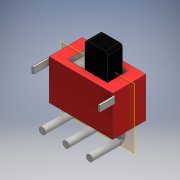
# Autodesk Inventor part: 5MS1S102AM6QE
Saved by Autodesk Inventor 2016 (Build 200138000, 138)
## iProperties
Created: 2018-08-01
Part Number: 5MS1S102AM6QE
Material: Generic
Document SubType Name: Modeling
Designer: Luke
Density: 1 g/cm^3
Appearance: Default
Author: Luke
Autodesk Inventor part; units mm, degrees
ref_plane "YZ Plane" through (0, 0, 0) normal (1, 0, 0) x (0, 1, 0)
sketch "Sketch1" plane through (0, 0, 0) normal (0, 0, 1) x (1, 0, 0)
  line L0 (0, 0) -> (12.7, 0)
  line L1 (12.7, 0) -> (12.7, 6.6)
  line L2 (12.7, 6.6) -> (0, 6.6)
  line L3 (0, 6.6) -> (0, 0)
  dimension "d0" = 12.7
  dimension "d1" = 6.6
  constraints: 8 end point, 2 parallel, 1 horizontal, 1 perpendicular
  measures "d0" distance of L1.end L2.end
  measures "d1" distance of L0.end L1.end
extrude "Extrusion1" add sketch "Sketch1" along normal blind 8
sketch "Sketch2" plane through (0, 0, 0) normal (0, -1, 0) x (1, 0, 0)
  line L0 (0, 0) -> (12.7, 0) construction
  line L1 (12.7, 0) -> (12.7, 8) construction
  line L2 (0, 8) -> (12.7, 8) construction
  line L3 (0, 0) -> (0, 8) construction
  line L4 (0, 0) -> (12.7, 0) construction
  line L5 (6.35, 0) -> (6.35, 8) construction
  line L6 (0, 8) -> (12.7, 8) construction
  line L7 (13.135, 7.585) -> (12.775, 7.585)
  line L8 (12.775, 7.585) -> (12.775, 6.415)
  line L9 (12.775, 6.415) -> (13.135, 6.415)
  line L10 (13.135, 6.415) -> (13.135, 7.585)
  line L11 (13.135, 7.585) -> (12.775, 6.415) construction
  line L12 (12.775, 7.585) -> (13.135, 6.415) construction
  circle A0 centre (6.35, -2.53) radius 0.635
  circle A1 centre (11.05, -2.53) radius 0.635
  circle A2 centre (1.65, -2.53) radius 0.635
  line L13 (11.05, -2.53) -> (6.35, -2.53) construction
  line L14 (6.35, -2.53) -> (1.65, -2.53) construction
  line L15 (-0.435, 7.585) -> (-0.075, 7.585)
  line L16 (-0.075, 7.585) -> (-0.075, 6.415)
  line L17 (-0.075, 6.415) -> (-0.435, 6.415)
  line L18 (-0.435, 6.415) -> (-0.435, 7.585)
  point P0 (12.955, 7)
  dimension "d4" = 1.17
  dimension "d5" = 0.36
  dimension "d6" = 6.605
  dimension "d7" = 1.27
  dimension "d8" = 1.27
  dimension "d9" = 1.27
  dimension "d10" = 9.53
  dimension "d11" = 4.7
  dimension "d12" = 4.7
  dimension "d13" = 1
  constraints: 26 end point, 4 midpoint, 4 symmetric about line, 3 centre point, 3 equal length, 2 horizontal, 1 perpendicular, 1 point on line
  measures "d4" distance of L9.end L7.start
  measures "d5" distance of L8.end L9.end
  measures "d6" distance from line of L5 point (12.955, 7)
  measures "d7" diameter of A0
  measures "d8" diameter of A1
  measures "d9" diameter of A2
  measures "d10" vertical distance of point (12.955, 7) L13.start
  measures "d11" distance of L13.end L13.start
  measures "d12" distance of L14.end L13.end
  measures "d13" distance from line of L2 point (12.955, 7)
extrude "Extrusion2" add sketch "Sketch2" along normal blind 3
ref_plane "Work Plane1" through (0, 2.6, 0) normal (0, 1, 0) x (1, 0, 0)
sketch "Sketch3" plane through (11.05, 0, -2.53) normal (0, 1, 0) x (1, 0, 0)
  circle A0 centre (0, 0) radius 0.635 projected
  circle A1 centre (-4.7, 0) radius 0.635 projected
  circle A2 centre (-9.4, 0) radius 0.635 projected
  point P0 (-11.05, -2.53)
extrude "Extrusion3" add sketch "Sketch3" along normal up to surface (2.6 mm away)
sketch "Sketch4" plane through (0, 0, 0) normal (0, 0, -1) x (-1, 0, 0)
  line L0 (-6.985, 2.6) -> (-5.715, 2.6) projected
  line L1 (-6.35, 2.6) -> (-6.35, 3.235) construction
  circle A0 centre (-6.35, 3.235) radius 0.635
  point P0 (0, 0)
  dimension "d19" = 0.635
  constraints: 2 end point, 1 coincident, 1 midpoint, 1 vertical, 1 vertical alignment, 2 other
  measures "d19" distance of L1.start L1.end
extrude "Extrusion4" add sketch "Sketch4" along normal blind 1.895
sketch "Sketch5" plane through (0, 0, -1.895) normal (0, 0, -1) x (-1, 0, 0)
  arc A0 (-5.715, 3.235) -> (-6.35, 2.6) centre (-6.35, 3.235) ccw construction
  arc A1 (-5.715, 3.235) -> (-6.35, 2.6) centre (-6.35, 3.235) ccw projected
  arc A2 (-6.35, 2.6) -> (-5.715, 3.235) centre (-6.35, 3.235) ccw projected
  point P0 (0, 0)
  constraints: 1 coincident
ref_plane "Work Plane2" through (6.35, 3.235, -1.895) normal (1, 0, 0) x (0, 0, -1)
sketch "Sketch6" plane through (6.35, 3.235, -1.895) normal (1, 0, 0) x (0, 0, -1)
  line L0 (0.635, -0.635) -> (0, -0.635) construction
  line L1 (0, -0.635) -> (0.635, -0.635) construction
  line L2 (0, -0.635) -> (0, 0) construction
  arc A0 (0.635, -0.635) -> (0, 0) centre (0, -0.635) ccw
  point P0 (-1.895, -3.235)
  constraints: 2 point on circle, 1 centre point, 1 coincident
sweep "Sweep1" add profiles "Sketch5" path "Sketch6"
pattern_linear "Rectangular Pattern1" count 3 spacing 4.7 along (-1, 0, 0) of "Sweep1", "Extrusion4" first direction both ways yes
sketch "Sketch7" plane through (-0.435, 0, 7.585) normal (0, 0, 1) x (1, 0, 0)
  line L0 (0.36, 0) -> (0, 0) projected
  line L1 (0.435, 0) -> (13.135, 0) projected
  line L2 (13.135, 0) -> (13.135, 6.6) projected
  line L3 (13.135, 6.6) -> (0.435, 6.6) projected
  line L4 (0.435, 6.6) -> (0.435, 0) projected
  line L5 (0.36, 0) -> (0.36, -3) projected
  line L6 (0.36, 0) -> (0.435, 0)
  line L7 (0, 0) -> (0.435, 0.2)
  line L8 (0.435, 6.6) -> (0.435, 0) projected
  dimension "d27" = 0.2
  constraints: 4 end point, 1 perpendicular, 1 point on line
  measures "d27" distance of L8.end L7.end
extrude "Extrusion5" add sketch "Sketch7" against normal up to surface (1.17 mm away) contours L0 L7 L4 L6
mirror "Mirror1" about plane through (6.35, 3.235, -1.895) normal (1, 0, 0) of "Extrusion5"
ref_plane "Work Plane3" through (0, 3.3, 0) normal (0, -1, 0) x (1, 0, 0)
sketch "Sketch9" plane through (0, 0, 8) normal (0, 0, 1) x (1, 0, 0)
  line L0 (15.849, 3.3) -> (-3.149, 3.3) projected
  line L1 (2.35, 5.3) -> (10.35, 5.3)
  line L2 (10.35, 5.3) -> (10.35, 1.3)
  line L3 (10.35, 1.3) -> (2.35, 1.3)
  line L4 (2.35, 1.3) -> (2.35, 5.3)
  line L5 (0, 0) -> (12.7, 0) construction
  line L6 (12.7, 0) -> (12.7, 6.6) construction
  line L7 (12.7, 6.6) -> (0, 6.6) construction
  line L8 (0, 6.6) -> (0, 0) construction
  line L9 (12.7, 6.6) -> (0, 6.6) construction
  line L10 (6.35, 6.6) -> (6.35, 0) construction
  line L11 (0, 0) -> (12.7, 0) construction
  dimension "d30" = 8
  dimension "d31" = 4
  constraints: 10 end point, 2 midpoint, 2 parallel, 1 horizontal, 1 perpendicular, 2 other
  measures "d30" distance of L1.start L1.end
  measures "d31" distance of L1.end L2.end
extrude "Extrusion6" cut sketch "Sketch9" against normal blind 1
sketch "Sketch10" plane through (0, 0, 7) normal (0, 0, 1) x (1, 0, 0)
  line L0 (2.35, 5.3) -> (10.35, 5.3) projected
  line L1 (2.35, 1.3) -> (2.35, 5.3) projected
  line L2 (10.35, 1.3) -> (2.35, 1.3) projected
  line L3 (10.35, 5.3) -> (10.35, 1.3) projected
  line L4 (9.85, 4.8) -> (5.35, 4.8)
  line L5 (5.35, 4.8) -> (5.35, 1.8)
  line L6 (5.35, 1.8) -> (9.85, 1.8)
  line L7 (9.85, 1.8) -> (9.85, 4.8)
  line L8 (15.849, 3.3) -> (-3.149, 3.3) construction
  point P0 (0, 0)
  dimension "d34" = 4.5
  dimension "d35" = 0.5
  dimension "d36" = 0.5
  constraints: 8 end point, 2 parallel, 1 horizontal, 1 perpendicular, 1 other
  measures "d34" distance of L4.start L4.end
  measures "d35" distance between parallel lines of L3 L7
  measures "d36" distance between parallel lines of L4 L0
extrude "Extrusion7" add sketch "Sketch10" along normal blind 5.72 contours L7 L6 L5 L4
fillet "Fillet1" radius 0.5 2 edges at (9.85, 3.3, 12.72) (5.35, 3.3, 12.72)
equation "\"d8\" = d7"
equation "\"d9\" = d7"
equation "\"d12\" = d11"
equation "\"d36\" = d35"
body "Solid1"
